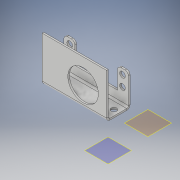
# Autodesk Inventor part: HSmount
Saved by Autodesk Inventor 2017 (Build 210142000, 142)
## iProperties
Created: 2017-02-21
Part Number: HSmount
Material: Generic
Document SubType Name: Sheet Metal
Designer: kingb
Density: 1 g/cm^3
Sheet Metal Rule: Default
Appearance: Default
Flat Pattern Width: 6.0325 cm
Flat Pattern Length: 8.88554 cm
Flat Pattern Area: 53.602 cm^2
Sheet Metal Width: 2.375 in
Sheet Metal Length: 3.498 in
Sheet Metal Area: 8.308 in^2
Mass: 6.04176 g
Surface Area: 84.401 cm^2
Volume: 6.04176 cm^3
Author: kingb
Autodesk Inventor part; units mm, degrees
ref_plane "YZ Plane" through (0, 0, 0) normal (1, 0, 0) x (0, 1, 0)
ref_plane "Work Plane1" through (-25.7458, -64.4152, -12.319) normal (0, -1, 0) x (0, 0, -1)
ref_plane "Work Plane2" through (0, 0, 0) normal (0, 0, 1) x (1, 0, 0)
sketch "Sketch1" plane through (0, 0, 0) normal (0, 0, 1) x (1, 0, 0)
  line L0 (-0.4093, 18.5158) -> (-5.7433, 18.5158) projected
  line L1 (-5.7433, -1.2962) -> (-5.7433, 18.5158) projected
  line L2 (-45.7483, 18.5158) -> (-51.0823, 18.5158) projected
  line L3 (-45.7483, 18.5158) -> (-45.7483, -1.2962) projected
  line L4 (-5.7433, 18.5158) -> (4.4167, 18.5158)
  line L5 (4.4167, 18.5158) -> (4.4167, -11.9642)
  line L6 (-45.7483, 18.5158) -> (-55.9083, 18.5158)
  line L7 (-55.9083, 18.5158) -> (-55.9083, -11.9642)
  line L8 (-55.9083, -11.9642) -> (4.4167, -11.9642)
  line L9 (-5.7433, -1.2962) -> (-45.7483, -1.2962)
  point P0 (0, 0)
  dimension "d0" = 10.16
  dimension "d1" = 30.48
  dimension "d2" = 10.16
  constraints: 12 end point, 2 perpendicular, 2 point on line, 1 parallel, 1 vertical
  measures "d0" distance of L0.end L4.end
  measures "d1" distance of L4.end L5.end
  measures "d2" distance of L2.start L6.end
extrude "Extrusion1" add sketch "Sketch1" along normal blind 1.5875
fillet "Corner Round1" radius 3.175 4 edges at (4.4167, 18.5158, 0.7937) (-5.7433, 18.5158, 0.7937) (-45.7483, 18.5158, 0.7937) (-55.9083, 18.5158, 0.7937)
sketch "Sketch2" plane through (4.4167, -10.3767, 0) normal (0, -1, 0) x (1, 0, 0)
  line L0 (-60.325, 0) -> (0, 0)
  line L1 (0, 0) -> (0, 16.9037)
  line L2 (0, 16.9037) -> (-60.325, 16.9037)
  line L3 (-60.325, 16.9037) -> (-60.325, 0)
  constraints: 6 end point, 1 horizontal, 1 perpendicular, 1 vertical
edge flange "Flange1" height 16.9037 angle 90 thickness 1.5875 bend radius 1.5875 thickness toward (0, -1, 0) relief straight relief width 1.5875 relief depth 0.7937 edges at (-25.7458, -11.9642, 1.5875) wall of the first edge with corners at (-55.9083, -10.3767, 0) (4.4167, -10.3767, 0) (4.4167, -10.3767, 16.9037) (-55.9083, -10.3767, 16.9037)
bend "Bend1"
corner "Corner1"
sketch "Sketch4" plane through (0, 0, 0) normal (0, 0, -1) x (-1, 0, 0)
  arc A0 (-0.8607, 1.809) -> (-0.8607, 5.4793) centre (1.057, 3.6441) ccw projected
  arc A1 (-0.8607, 11.7404) -> (-0.8607, 15.4107) centre (1.057, 13.5755) ccw projected
  arc A2 (52.3523, 15.4107) -> (52.3523, 11.7404) centre (50.4346, 13.5755) ccw projected
  arc A3 (52.3523, 5.4793) -> (52.3523, 1.809) centre (50.4346, 3.6441) ccw projected
  arc A4 (52.3523, 1.809) -> (52.3523, 5.4793) centre (50.4346, 3.6441) ccw
  arc A5 (52.3523, 11.7404) -> (52.3523, 15.4107) centre (50.4346, 13.5755) ccw
  arc A6 (-0.8607, 5.4793) -> (-0.8607, 1.809) centre (1.057, 3.6441) ccw
  arc A7 (-0.8607, 15.4107) -> (-0.8607, 11.7404) centre (1.057, 13.5755) ccw
  point P0 (0, 0)
  constraints: 8 point on circle, 4 centre point, 4 concentric
extrude "Extrusion2" cut sketch "Sketch4" against normal up to surface (1.5875 mm away)
ref_plane "Work Plane4" through (4.4167, -10.3767, 3.175) normal (0, 1, 0) x (1, 0, 0)
sketch "Sketch8" plane through (4.4167, -10.3767, 3.175) normal (0, 1, 0) x (1, 0, 0)
  line L0 (12.7, -13.7287) -> (-73.025, -13.7287) projected
  line L1 (0, 0) -> (-0.1034, -13.7287)
  line L2 (-60.325, 0) -> (0, 0) projected
  line L3 (-60.325, 0) -> (-60.325, -13.7287)
  line L4 (-3.175, 1.5875) -> (-6.985, 1.5875) projected
  line L5 (-5.08, 1.5875) -> (-5.08, -6.8643)
  line L6 (-5.08, -6.8643) -> (0, -6.8644)
  line L7 (0, -13.7287) -> (0, 0) projected
  line L8 (-53.34, 1.5875) -> (-57.15, 1.5875) projected
  line L9 (-55.245, 1.5875) -> (-55.245, -6.8644)
  point P0 (-4.4167, 3.175)
  constraints: 10 end point, 3 midpoint, 2 vertical, 1 perpendicular, 1 point on line
ref_plane "Work Plane3" through (4.4167, -11.9642, 3.175) normal (0, -1, 0) x (1, 0, 0)
sketch "Sketch9" plane through (4.4167, -11.9642, 3.175) normal (0, -1, 0) x (1, 0, 0)
  line L0 (12.7, 13.7287) -> (-73.025, 13.7287) projected
  line L1 (0, 13.7287) -> (-60.325, 13.7287)
  line L2 (-60.325, 13.7287) -> (-60.325, 18.8087)
  line L3 (-60.325, 18.8087) -> (0, 18.8087)
  line L4 (0, 18.8087) -> (0, 13.7287)
  line L5 (-60.325, 13.7287) -> (-60.325, 0) projected
  line L6 (0, 13.7287) -> (0, 0) projected
  point P0 (-4.4167, -3.175)
  dimension "d57" = 5.08
  constraints: 8 end point, 2 collinear, 2 parallel, 1 horizontal, 1 perpendicular, 1 point on line
  measures "d57" distance of L3.end L1.start
extrude "Extrusion6" add sketch "Sketch9" against normal blind 1.5875
sketch "Sketch11" plane through (4.4167, -11.9642, 20.3962) normal (0, 0, 1) x (1, 0, 0)
  line L0 (-60.325, 0) -> (0, 0)
  line L1 (0, 0) -> (0, 41.91)
  line L2 (0, 41.91) -> (-60.325, 41.91)
  line L3 (-60.325, 41.91) -> (-60.325, 0)
  constraints: 6 end point, 1 horizontal, 1 perpendicular, 1 vertical
edge flange "Flange4" height 41.91 angle 90 thickness 1.5875 bend radius 1.5875 thickness toward (0, 0, 1) relief straight relief width 1.5875 relief depth 0.7937 edges at (-25.7458, -10.3767, 21.9837) wall of the first edge with corners at (-55.9083, -11.9642, 20.3962) (4.4167, -11.9642, 20.3962) (4.4167, 29.9458, 20.3962) (-55.9083, 29.9458, 20.3962)
bend "Bend4"
corner "Corner4"
hole "Hole1" at (-0.6633, -10.3767, 10.0393) at (-50.8283, -10.3767, 10.0393) direction (0, -1, 0) diameter 5.1308 end through all
sketch "Sketch12" plane through (4.4167, 29.9458, 20.3962) normal (0, 0, -1) x (-1, 0, 0)
  line L0 (21.971, 0.0162) -> (21.971, -22.9454)
  line L1 (60.325, 0) -> (60.325, -38.735) projected
  line L2 (0, 0) -> (0, -38.735) projected
  point P0 (4.4167, -29.9458)
  dimension "d65" = 22.9616
  dimension "d74" = 21.971
  constraints: 2 end point, 1 vertical
  measures "d65" distance of L0.start L0.end
  measures "d74" distance from line of L2 L0.start
hole "Hole2" at (-17.5543, 7.0004, 20.3962) direction (0, 0, 1) diameter 28.575 end through all
equation "\"d63\" = Thickness"
equation "\"d72\" = Thickness"
equation "\"d6\" = BendReliefWidth"
equation "\"d7\" = BendReliefDepth"
equation "\"d8\" = MinimumRemnant"
equation "\"d9\" = BendRadius"
equation "\"d12\" = BendRadius"
equation "\"d13\" = CornerReliefSize"
equation "\"d14\" = GapSize"
equation "\"d15\" = JacobiRadiusSize"
equation "\"d47\" = BendReliefWidth"
equation "\"d48\" = BendReliefDepth"
equation "\"d49\" = MinimumRemnant"
equation "\"d50\" = BendRadius"
equation "\"d53\" = BendRadius"
equation "\"d54\" = CornerReliefSize"
equation "\"d55\" = GapSize"
equation "\"d56\" = JacobiRadiusSize"
equation "\"BendRadius\" = Thickness"
equation "\"BendReliefWidth\" = Thickness"
equation "\"BendReliefDepth\" = 0.5 * Thickness"
equation "\"CornerReliefSize\" = 4 * Thickness"
equation "\"MinimumRemnant\" = 2 * Thickness"
equation "\"TransitionRadius\" = BendRadius"
equation "\"JacobiRadiusSize\" = Thickness"
equation "\"GapSize\" = Thickness"
equation "\"Thickness\" = 1.5875"
body "Solid1"
